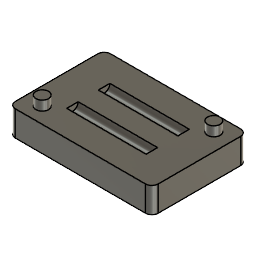
Ecoflex_Pad_Mold_Bottom (Autodesk Fusion 360 design; units mm, degrees)
part number: 2026-08-12-16-44-17-815
Autodesk Fusion 360 part; units mm, degrees
sketch "草图1" plane through (0, 0, 0) normal (0, 0, 1) x (1, 0, 0)
  line L0 (22.5, -15) -> (-22.5, -15)
  line L1 (-22.5, -15) -> (-22.5, 15)
  line L2 (-22.5, 15) -> (22.5, 15)
  line L3 (22.5, 15) -> (22.5, -15)
  line L4 (22.5, -15) -> (-22.5, 15) construction
  line L5 (-22.5, -15) -> (22.5, 15) construction
  dimension "d27" = 45
  dimension "d28" = 30
  constraint horizontal L0
  constraint perpendicular L0 L1
  constraint parallel L0 L2
  constraint parallel L1 L3
  constraint coincident L4 origin
  constraint coincident L5 origin
  measures "d27" distance of L1.end L2.end
  measures "d28" distance of L0.start L2.end
extrude "拉伸1" add sketch "草图1" along normal blind 8
sketch "草图2" plane through (0, 0, 0) normal (1, 0, 0) x (0, 1, 0)
  circle A0 centre (5, 8) radius 1.8
  dimension "d31" = 3.6
  measures "d31" diameter of A0
extrude "拉伸2" cut sketch "草图2" along normal blind 12.5 and the other way blind 12.5
mirror "镜像1" about plane through (0, 0, 0) normal (0, 1, 0) of "拉伸2"
sketch "草图3" plane through (0, 0, 8) normal (0, 0, 1) x (-1, 0, 0)
  line L0 (12.5, 6.8) -> (12.5, 3.2)
  line L1 (12.5, 3.2) -> (-12.5, 3.2)
  line L2 (-12.5, 3.2) -> (-12.5, 6.8)
  line L3 (-12.5, 6.8) -> (12.5, 6.8)
  line L4 (12.5, -3.2) -> (12.5, -6.8)
  line L5 (12.5, -6.8) -> (-12.5, -6.8)
  line L6 (-12.5, -6.8) -> (-12.5, -3.2)
  line L7 (-12.5, -3.2) -> (12.5, -3.2)
  line L8 (-22.5, -15) -> (22.5, -15)
  line L9 (22.5, -15) -> (22.5, 15)
  line L10 (22.5, 15) -> (-22.5, 15)
  line L11 (-22.5, 15) -> (-22.5, -15)
  circle A0 centre (17, 10) radius 2
  circle A1 centre (-17, -10) radius 2
  dimension "d38" = 4
  dimension "d39" = 4
  measures "d38" diameter of A0
  measures "d39" diameter of A1
extrude "拉伸3" add sketch "草图3" along normal blind 3 contours A0 | A1
fillet "圆角1" radius 2 4 edges at (-22.5, -15, 4) (-22.5, 15, 4) (22.5, 15, 4) (22.5, -15, 4)
equation "Catheter_Diameter = 2.4 mm" comment "Flexible spring catheter outer diameter"
equation "Catheter_Assembly_Clearance = 0.2 mm" comment "Initial diametral assembly clearance between catheter and Ecoflex liner"
equation "Clamp_Groove_Diameter = 3.6 mm" comment "Hard clamp circular groove diameter"
equation "Pad_Outer_Diameter = Clamp_Groove_Diameter" comment "Ecoflex liner outer diameter driven by clamp groove"
equation "Pad_Outer_Radius = Pad_Outer_Diameter / 2" comment "Ecoflex liner outer radius"
equation "Pad_Inner_Diameter = Catheter_Diameter + Catheter_Assembly_Clearance" comment "Ecoflex liner inner diameter"
equation "Pad_Inner_Radius = Pad_Inner_Diameter / 2" comment "Ecoflex liner inner radius"
equation "Pad_Radial_Thickness = ( Pad_Outer_Diameter - Pad_Inner_Diameter ) / 2" comment "Nominal radial thickness of Ecoflex liner"
equation "Pad_Length = 25 mm" comment "Effective Ecoflex liner length"
equation "Mold_Length = 45 mm" comment "Overall mold length along X"
equation "Mold_Width = 30 mm" comment "Overall mold width along Y"
equation "Bottom_Mold_Thickness = 8 mm" comment "Bottom mold plate thickness"
equation "Top_Mold_Thickness = 6 mm" comment "Top mold plate thickness"
equation "Top_Mold_Base_Z = Bottom_Mold_Thickness" comment "Assembly Z height of top mold bottom parting face"
equation "Pad_Cavity_Offset_Y = 5 mm" comment "Centerline offset of the two cavities from mold center"
equation "Alignment_Pin_Diameter = 4 mm" comment "Printed alignment pin diameter on bottom mold"
equation "Alignment_Pin_Height = 3 mm" comment "Alignment pin height"
equation "Alignment_Hole_Diameter = 4.4 mm" comment "Alignment blind-hole diameter on top mold"
equation "Alignment_Hole_Depth = 3.4 mm" comment "Alignment blind-hole depth"
equation "Alignment_Pin_Offset_X = 17 mm" comment "Absolute X coordinate magnitude of alignment pins"
equation "Alignment_Pin_Offset_Y = 10 mm" comment "Absolute Y coordinate magnitude of alignment pins"
equation "Overflow_Channel_Width = 1 mm" comment "Optional V1 overflow-channel width; retained but not used in recommended V1"
equation "Overflow_Channel_Depth = 0.4 mm" comment "Optional V1 overflow-channel depth; retained but not used in recommended V1"
equation "Overflow_Well_Diameter = 6 mm" comment "Optional overflow-well diameter; retained but not used in recommended V1"
equation "Overflow_Well_Depth = 1 mm" comment "Optional overflow-well depth; retained but not used in recommended V1"
equation "Mold_Outer_Fillet = 2 mm" comment "External handling-edge fillet radius"
equation "d27 = Mold_Length"
equation "d28 = Mold_Width"
equation "d29 = Bottom_Mold_Thickness"
equation "d31 = Pad_Outer_Diameter"
equation "d32 = Pad_Length / 2"
equation "d34 = Pad_Length / 2"
equation "d38 = Alignment_Pin_Diameter"
equation "d43 = Mold_Outer_Fillet"
